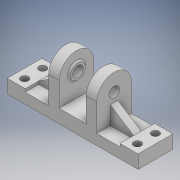
# Autodesk Inventor part: parte_3_base
Saved by Autodesk Inventor 2018 (Build 220112000, 112)
## iProperties
Created: 2018-04-07
Part Number: parte_3_base
Material: Generic
Document SubType Name: Modeling
Designer: Francisco
Density: 1 g/cm^3
Appearance: Default
Author: Francisco
Autodesk Inventor part; units mm, degrees
ref_plane "YZ Plane" through (0, 0, 0) normal (1, 0, 0) x (0, 1, 0)
ref_plane "XZ Plane" through (0, 0, 0) normal (0, 1, 0) x (-1, 0, 0)
ref_plane "XY Plane" through (0, 0, 0) normal (0, 0, 1) x (1, 0, 0)
sketch "Sketch1" plane through (0, 0, 0) normal (0, 0, 1) x (1, 0, 0)
  line L0 (-87, 23) -> (87, 23)
  line L1 (87, 23) -> (87, -23)
  line L2 (87, -23) -> (-87, -23)
  line L3 (-87, -23) -> (-87, 23)
  line L4 (-87, 23) -> (87, -23) construction
  line L5 (87, 23) -> (-87, -23) construction
  circle A0 centre (-75, -12) radius 5
  circle A1 centre (-75, 12) radius 5
  circle A2 centre (75, -12) radius 5
  circle A3 centre (75, 12) radius 5
  point P0 (0, 0)
  dimension "d0" = 174
  dimension "d1" = 46
  dimension "d3" = 10
  dimension "d6" = 24
  dimension "d9" = 150
  dimension "d12" = 11
  dimension "d13" = 12
  constraints: 12 end point, 4 centre point, 2 horizontal, 2 midpoint, 2 parallel, 1 perpendicular, 1 vertical, 6 other
  measures "d0" distance of L1.end L2.end
  measures "d1" distance of L0.end L1.end
  measures "d3" diameter of A0
  measures "d6" distance of A0.centre A1.centre
  measures "d9" distance of A0.centre A2.centre
  measures "d12" distance from line of L2 A0.centre
  measures "d13" distance from line of L3 A0.centre
extrude "Extrusion1" add sketch "Sketch1" along normal blind 18
sketch "Sketch2" plane through (0, 0, 18) normal (0, 0, 1) x (1, 0, 0)
  line L0 (-87, -23) -> (87, -23) projected
  line L1 (32, 23) -> (63, 23)
  line L2 (63, 23) -> (63, -23)
  line L3 (63, -23) -> (32, -23)
  line L4 (32, -23) -> (32, 23)
  line L5 (87, -23) -> (87, 23) projected
  point P0 (0, 0)
  dimension "d16" = 24
  dimension "d17" = 55
  dimension "d18" = 46
  constraints: 8 end point, 2 parallel, 1 horizontal, 1 perpendicular, 1 point on line
  measures "d16" distance between parallel lines of L5 L2
  measures "d17" distance between parallel lines of L5 L4
  measures "d18" distance of L1.end L2.end
extrude "Extrusion2" cut sketch "Sketch2" against normal blind 4
sketch "Sketch3" plane through (0, 0, 0) normal (0, 1, 0) x (-1, 0, 0)
  line L0 (-32, 18) -> (87, 18) projected
  line L1 (-32, 18) -> (-32, 14) projected
  line L2 (-32, 14) -> (-63, 14) projected
  line L3 (-87, 18) -> (-63, 18) projected
  line L4 (-16, 57) -> (-32, 57)
  line L5 (-32, 57) -> (-32, 73)
  line L6 (-32, 73) -> (-18, 73)
  line L7 (-18, 73) -> (-18, 60)
  line L8 (-18, 60) -> (-16, 60)
  line L9 (-16, 60) -> (-16, 57)
  line L10 (-3, 50) -> (-39, 50) construction
  line L11 (87, 0) -> (-87, 0) construction
  line L12 (-63, 14) -> (-63, 18) projected
  line L13 (-32, 14) -> (-32, 18) projected
  point P0 (0, 0)
  point P1 (-32, 16)
  dimension "d21" = 50
  dimension "d22" = 14
  dimension "d23" = 46
  dimension "d24" = 16
  dimension "d25" = 14
  dimension "d26" = 3
  constraints: 14 end point, 5 perpendicular, 2 horizontal, 1 collinear, 1 midpoint
  measures "d21" distance between parallel lines of L11 L10
  measures "d22" diameter of L4 L10
  measures "d23" diameter of L6 L10
  measures "d24" distance between parallel lines of L5 L9
  measures "d25" distance between parallel lines of L5 L7
  measures "d26" distance between parallel lines of L4 L8
revolve "Revolution1" add sketch "Sketch3" angle 360 about axis through (3, 0, 50) along (1, 0, 0)
sketch "Sketch4" plane through (0, 0, 18) normal (0, 0, 1) x (1, 0, 0)
  line L0 (32, 23) -> (-87, 23) projected
  line L1 (87, -23) -> (-87, -23) projected
  line L2 (18, 23) -> (32, 23)
  line L3 (32, 23) -> (32, -23)
  line L4 (32, -23) -> (18, -23)
  line L5 (18, -23) -> (18, 23)
  line L6 (32, -23) -> (32, 23) projected
  point P0 (0, 0)
  dimension "d28" = 14
  constraints: 8 end point, 3 equal length, 2 point on line, 1 horizontal, 1 perpendicular
  measures "d28" distance between parallel lines of L3 L5
extrude "Extrusion3" add sketch "Sketch4" along normal up to next
fillet "Fillet1" radius 2 1 edges at (18, 0, 40)
sketch "Sketch8" plane through (0, 0, 0) normal (0, 1, 0) x (-1, 0, 0)
  line L0 (-63, 18) -> (-32, 38)
  line L1 (-32, 14) -> (-32, 50) projected
  line L2 (-63, 18) -> (-63, 14) projected
  line L3 (-32, 14) -> (-32, 50) projected
  line L4 (-32, 50) -> (-18, 50) projected
  line L5 (-18, 18) -> (-18, 50) projected
  line L6 (87, 18) -> (-18, 18) projected
  line L7 (87, 0) -> (87, 18) projected
  line L8 (-87, 0) -> (87, 0) projected
  line L9 (-87, 0) -> (-87, 18) projected
  line L10 (-63, 18) -> (-87, 18) projected
  line L11 (-63, 18) -> (-63, 14) projected
  line L12 (-63, 14) -> (-32, 14) projected
  point P0 (0, 0)
  dimension "d35" = 12
  constraints: 2 end point, 1 vertical alignment
  measures "d35" distance of L0.end L1.end
extrude "Rib1" add sketch "Sketch8" along normal mid plane 10 rib yes fills toward (-47.4729, 27.958) open curves L0
mirror "Mirror1" about plane through (0, 0, 0) normal (1, 0, 0) of "Extrusion2", "Revolution1", "Extrusion3", "Fillet1", "Rib1"
ref_plane "Work Plane2" through (0, 0, 0) normal (1, 0, 0) x (0, 1, 0)
body "Solid1"
